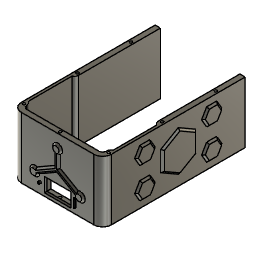
teslacoil assembly v1 (Autodesk Fusion 360 archive; units mm, degrees)
design "walls"
Autodesk Fusion 360 part; units mm, degrees
(part 1 of 3)
sketch "Sketch1" plane through (0, 0, 0) normal (0, 0, 1) x (1, 0, 0)
  line L0 (41.5, 125) -> (-41.5, 125)
  arc A0 (-41.5, 125) -> (-51.5, 115) centre (-41.5, 115) ccw
  line L1 (-51.5, 115) -> (-51.5, -130)
  arc A1 (51.5, 115) -> (41.5, 125) centre (41.5, 115) ccw
  line L2 (51.5, -130) -> (51.5, 115)
  line L3 (-41.5, -140) -> (41.5, -140)
  arc A2 (41.5, -140) -> (51.5, -130) centre (41.5, -130) ccw
  arc A3 (-51.5, -130) -> (-41.5, -140) centre (-41.5, -130) ccw
  line L4 (0, 125) -> (0, 122)
  line L5 (-51.5, 115) -> (-48.5, 115)
  circle A4 centre (-48.5, 115) radius 1.5
  circle A5 centre (0, 122) radius 1.5
  circle A6 centre (-48.5, -7.5) radius 1.5
  circle A7 centre (-48.5, 53.75) radius 1.5
  circle A8 centre (-48.5, -130) radius 1.5
  circle A9 centre (-48.5, -68.75) radius 1.5
  circle A10 centre (-48.5, -7.5) radius 1.5
  circle A11 centre (48.5, 115) radius 1.5
  circle A12 centre (48.5, 53.75) radius 1.5
  circle A13 centre (48.5, -7.5) radius 1.5
  circle A14 centre (48.5, -68.75) radius 1.5
  circle A15 centre (48.5, -130) radius 1.5
  line L6 (0, -140) -> (0, -137)
  circle A16 centre (0, -137) radius 1.5
  arc A17 (-45.5, -130) -> (-41.5, -134) centre (-41.5, -130) ccw
  line L7 (-41.5, -134) -> (41.5, -134)
  arc A18 (41.5, -134) -> (45.5, -130) centre (41.5, -130) ccw
  arc A19 (45.5, 115) -> (41.5, 119) centre (41.5, 115) ccw
  line L8 (41.5, 119) -> (-41.5, 119)
  line L9 (-48.5, -99.375) -> (-48.5, -75)
  line L10 (-48.5, -99.375) -> (-48.5, -125)
  line L11 (-45.5, 115) -> (-45.5, -75)
  line L12 (-45.5, -125) -> (-45.5, -130)
  line L13 (45.5, -130) -> (45.5, -125)
  line L14 (45.5, -75) -> (45.5, 115)
  line L15 (-48.5, -75) -> (-45.5, -75)
  line L16 (45.5, -75) -> (48.5, -75)
  line L17 (-48.5, -125) -> (-45.5, -125)
  line L18 (45.5, -125) -> (48.5, -125)
  line L19 (-48.5, -75) -> (-48.5, -125)
  line L20 (48.5, -75) -> (48.5, -125)
  arc A20 (-41.5, 119) -> (-45.5, 115) centre (-41.5, 115) ccw
  dimension "d1" = 3
  dimension "d3" = 3
  dimension "d4" = 3
  dimension "d5" = 3
  dimension "d7" = 3
  dimension "d8" = 3
  dimension "d9" = 3
  dimension "d10" = 3
  constraint midpoint L0 L4.start
  constraint perpendicular L0 L4
  constraint coincident L5.end A4.centre
  constraint coincident L4.end A5.centre
  constraint symmetric L4 A4 A11
  constraint symmetric L4 A7 A12
  constraint symmetric L4 A8 A15
  constraint symmetric L4 A9 A14
  constraint symmetric L4 A10 A13
  constraint midpoint L3 L6.start
  constraint perpendicular L3 L6
  constraint coincident L6.end A16.centre
  constraint perpendicular L10 L15
  constraint concentric A3 A17
  constraint concentric A2 A18
  constraint concentric A1 A19
  constraint tangent L7 A18
  constraint tangent A17 L7
  constraint tangent A17 L11
  constraint tangent A19 L13
  constraint tangent A18 L13
  constraint tangent A19 L8
  constraint collinear L11 L12
  constraint coincident L13.end L17
  constraint coincident L14.start L15
  constraint collinear L13 L14
  constraint collinear L15 L16
  constraint collinear L17 L18
  constraint symmetric L4 A19.start L11.start
  constraint symmetric L4 A19.end L8.end
  constraint symmetric L4 A19 A20
  measures "d1" distance of L4.start L4.end
  measures "d3" distance of A0.end L5.end
  measures "d4" diameter of A4
  measures "d5" diameter of A5
  measures "d7" diameter of A6
  measures "d8" diameter of A7
  measures "d9" distance of L6.start L6.end
  measures "d10" diameter of A16
extrude "Extrude1" add sketch "Sketch1" along normal blind 70
fillet "Fillet1" radius 5 4 edges at (45.5, -125, 35) (45.5, -75, 35) (-45.5, -75, 35) (-45.5, -125, 35)
sketch "Sketch2" plane through (0, 0, 70) normal (0, 0, 1) x (-1, 0, 0)
  arc A0 (45.5, 129.5826) -> (48.5, 125) centre (50.5, 129.5826) ccw
  line L0 (48.5, 125) -> (48.5, 75)
  arc A1 (48.5, 75) -> (45.5, 70.4174) centre (50.5, 70.4174) ccw
  line L1 (45.5, 70.4174) -> (45.5, -115)
  arc A2 (41.5, -119) -> (45.5, -115) centre (41.5, -115) ccw
  line L2 (41.5, -119) -> (-41.5, -119)
  arc A3 (-45.5, -115) -> (-41.5, -119) centre (-41.5, -115) ccw
  line L3 (-45.5, -115) -> (-45.5, 70.4174)
  arc A4 (-45.5, 70.4174) -> (-48.5, 75) centre (-50.5, 70.4174) ccw
  line L4 (-48.5, 75) -> (-48.5, 125)
  arc A5 (-48.5, 125) -> (-45.5, 129.5826) centre (-50.5, 129.5826) ccw
  line L5 (-45.5, 129.5826) -> (-45.5, 130)
  arc A6 (-41.5, 134) -> (-45.5, 130) centre (-41.5, 130) ccw
  line L6 (-41.5, 134) -> (41.5, 134)
  arc A7 (45.5, 130) -> (41.5, 134) centre (41.5, 130) ccw
  line L7 (45.5, 130) -> (45.5, 129.5826)
  circle A8 centre (48.5, -115) radius 1.5
  circle A9 centre (0, 137) radius 1.5
  circle A10 centre (0, -122) radius 1.5
  circle A11 centre (-48.5, 68.75) radius 1.5
  circle A12 centre (48.5, 130) radius 1.5
  circle A13 centre (-48.5, -115) radius 1.5
  circle A14 centre (-48.5, 130) radius 1.5
  circle A15 centre (48.5, 7.5) radius 1.5
  circle A16 centre (48.5, -53.75) radius 1.5
  circle A17 centre (-48.5, -53.75) radius 1.5
  circle A18 centre (-48.5, 7.5) radius 1.5
  circle A19 centre (48.5, 68.75) radius 1.5
  arc A20 (51.5, 130) -> (41.5, 140) centre (41.5, 130) ccw
  line L8 (41.5, 140) -> (-41.5, 140)
  arc A21 (-41.5, 140) -> (-51.5, 130) centre (-41.5, 130) ccw
  line L9 (-51.5, 130) -> (-51.5, -115)
  arc A22 (-51.5, -115) -> (-41.5, -125) centre (-41.5, -115) ccw
  line L10 (-41.5, -125) -> (41.5, -125)
  arc A23 (41.5, -125) -> (51.5, -115) centre (41.5, -115) ccw
  line L11 (51.5, -115) -> (51.5, 130)
  line L12 (48.5, -53.75) -> (48.5, 7.5)
  line L13 (-48.5, -53.75) -> (-48.5, 7.5)
  line L14 (48.5, -23.125) -> (-48.5, -23.125)
  line L15 (51.5, -23.125) -> (48.5, -23.125)
  line L16 (-48.5, -23.125) -> (-56, -23.125)
  constraint coincident A16.centre L12.start
  constraint coincident A15.centre L12.end
  constraint coincident A17.centre L13.start
  constraint coincident A18.centre L13.end
  constraint midpoint L12 L14.start
  constraint midpoint L13 L14.end
  constraint coincident L11 L15.start
  constraint perpendicular L12 L15
  constraint perpendicular L9 L16
extrude "Extrude2" cut sketch "Sketch2" against normal blind 80 contours L1 A2 L2 A3 L3 L9 A22 L10 A23 L11 L14 L15 L16
sketch "Sketch3" plane through (51.5, 0, 0) normal (1, 0, 0) x (0, 1, 0)
  line L0 (23.125, 0) -> (23.125, 70)
  line L1 (23.125, 70) -> (-130, 70)
  line L2 (-130, 70) -> (-130, 0)
  line L3 (-130, 0) -> (23.125, 0)
  line L4 (-53.4375, 70) -> (-53.4375, 0)
  line L5 (23.125, 35) -> (-130, 35)
  line L6 (-53.4375, 35) -> (-130, 70)
  line L7 (-53.4375, 35) -> (-130, 0)
  line L8 (-53.4375, 35) -> (23.125, 0)
  line L9 (-53.4375, 35) -> (23.125, 70)
  line L10 (-85.9452, 42.5) -> (-80.1717, 52.5)
  line L11 (-80.1717, 52.5) -> (-85.9452, 62.5)
  line L12 (-85.9452, 62.5) -> (-97.4923, 62.5)
  line L13 (-97.4923, 62.5) -> (-103.2658, 52.5)
  line L14 (-103.2658, 52.5) -> (-97.4923, 42.5)
  line L15 (-97.4923, 42.5) -> (-85.9452, 42.5)
  line L16 (-85.9452, 7.5) -> (-97.4923, 7.5)
  line L17 (-80.1717, 17.5) -> (-85.9452, 7.5)
  line L18 (-85.9452, 27.5) -> (-80.1717, 17.5)
  line L19 (-97.4923, 27.5) -> (-85.9452, 27.5)
  line L20 (-103.2658, 17.5) -> (-97.4923, 27.5)
  line L21 (-97.4923, 7.5) -> (-103.2658, 17.5)
  line L22 (-9.3827, 27.5) -> (-20.9298, 27.5)
  line L23 (-20.9298, 27.5) -> (-26.7033, 17.5)
  line L24 (-26.7033, 17.5) -> (-20.9298, 7.5)
  line L25 (-20.9298, 7.5) -> (-9.3827, 7.5)
  line L26 (-9.3827, 7.5) -> (-3.6092, 17.5)
  line L27 (-3.6092, 17.5) -> (-9.3827, 27.5)
  line L28 (-3.6092, 52.5) -> (-9.3827, 42.5)
  line L29 (-9.3827, 42.5) -> (-20.9298, 42.5)
  line L30 (-20.9298, 42.5) -> (-26.7033, 52.5)
  line L31 (-26.7033, 52.5) -> (-20.9298, 62.5)
  line L32 (-20.9298, 62.5) -> (-9.3827, 62.5)
  line L33 (-9.3827, 62.5) -> (-3.6092, 52.5)
  line L34 (-33.4375, 46.547) -> (-53.4375, 58.094)
  line L35 (-53.4375, 58.094) -> (-73.4375, 46.547)
  line L36 (-73.4375, 46.547) -> (-73.4375, 23.453)
  line L37 (-73.4375, 23.453) -> (-53.4375, 11.906)
  line L38 (-53.4375, 11.906) -> (-33.4375, 23.453)
  line L39 (-33.4375, 23.453) -> (-33.4375, 46.547)
  point P0 (-91.7188, 52.5)
  point P1 (-53.4375, 35)
  dimension "d18" = 10
  dimension "d19" = 20
  constraint midpoint L1 L4.start
  constraint midpoint L3 L4.end
  constraint midpoint L0 L5.start
  constraint midpoint L2 L5.end
  constraint midpoint L4 P1
  constraint coincident L1.end L2.start
  constraint coincident L2.end L3.start
  constraint coincident L0.start L3.end
  constraint coincident L0.end L1.start
  constraint midpoint L6 P0
  constraint symmetric L5 L10.start L18.start
  constraint symmetric L5 L10.end L17.start
  constraint symmetric L5 L11.end L16.start
  constraint symmetric L5 L12.end L16.end
  constraint symmetric L5 L13.end L20.start
  constraint symmetric L5 L14.end L19.start
  constraint symmetric L4 L10.start L29.end
  constraint symmetric L4 L10.end L30.end
  constraint symmetric L4 L11.end L31.end
  constraint symmetric L4 L12.end L32.end
  constraint symmetric L4 L13.end L28.start
  constraint symmetric L4 L14.end L28.end
  constraint symmetric L4 L16.start L24.end
  constraint symmetric L4 L16.end L25.end
  constraint symmetric L4 L17.start L23.end
  constraint symmetric L4 L18.start L22.end
  constraint symmetric L4 L19.start L22.start
  constraint symmetric L4 L20.start L26.end
  constraint coincident P1 L6.start
  measures "d18" distance of P0 L15
  measures "d19" distance of P1 L39
extrude "Extrude3" add sketch "Sketch3" along normal blind 2 contours L8 L23 L24 L25 L26 | L8 L22 L23 L26 L27 | L5 L8 L39 | L5 L9 L39 | L4 L7 L36 L37 | L4 L8 L38 L39 | L9 L28 L29 L30 L33 | L9 L30 L31 L32 L33 | L4 L6 L35 L36 | L5 L7 L36 | L5 L6 L36 | L4 L9 L34 L39 | L7 L18 L19 L20 L21 | L7 L16 L17 L18 L21 | L6 L10 L11 L12 L13 | L6 L10 L13 L14 L15
chamfer "Chamfer1" distance 2 angle 45 30 edges at (53.5, -63.4375, 52.3205) (53.5, -43.4375, 52.3205) (53.5, -33.4375, 35) (53.5, -43.4375, 17.6795) (53.5, -63.4375, 17.6795) (53.5, -73.4375, 35) (53.5, -91.7188, 42.5) (53.5, -83.0585, 57.5) (53.5, -100.379, 57.5) (53.5, -91.7188, 62.5) (53.5, -100.379, 47.5) (53.5, -100.379, 22.5) (53.5, -83.0585, 22.5) (53.5, -91.7188, 27.5) (53.5, -100.379, 12.5) (53.5, -91.7188, 7.5) (53.5, -83.0585, 12.5) (53.5, -83.0585, 47.5) (53.5, -15.1563, 62.5) (53.5, -6.496, 57.5) (53.5, -6.496, 47.5) (53.5, -15.1563, 42.5) (53.5, -23.8165, 47.5) (53.5, -23.8165, 57.5) (53.5, -23.8165, 22.5) (53.5, -23.8165, 12.5) (53.5, -15.1563, 7.5) (53.5, -6.496, 12.5) (53.5, -15.1563, 27.5) (53.5, -6.496, 22.5)
sketch "Sketch4" plane through (-51.5, 0, 0) normal (-1, 0, 0) x (0, -1, 0)
  line L0 (-23.125, 70) -> (-23.125, 0)
  line L1 (-23.125, 0) -> (130, 0)
  line L2 (130, 0) -> (130, 70)
  line L3 (130, 70) -> (-23.125, 70)
  line L4 (9.3827, 42.5) -> (20.9298, 42.5)
  line L5 (20.9298, 27.5) -> (26.7033, 17.5)
  line L6 (20.9298, 7.5) -> (9.3827, 7.5)
  line L7 (97.4923, 62.5) -> (103.2658, 52.5)
  line L8 (85.9452, 7.5) -> (97.4923, 7.5)
  line L9 (53.4375, 58.094) -> (33.4375, 46.547)
  line L10 (85.9452, 42.5) -> (80.1717, 52.5)
  line L11 (97.4923, 7.5) -> (103.2658, 17.5)
  line L12 (73.4375, 46.547) -> (53.4375, 58.094)
  line L13 (33.4375, 46.547) -> (33.4375, 23.453)
  line L14 (20.9298, 42.5) -> (26.7033, 52.5)
  line L15 (53.4375, 70) -> (53.4375, 0)
  line L16 (73.4375, 23.453) -> (73.4375, 46.547)
  line L17 (-23.125, 0) -> (130, 0)
  line L18 (53.4375, 35) -> (-23.125, 70)
  line L19 (53.4375, 11.906) -> (73.4375, 23.453)
  line L20 (9.3827, 7.5) -> (3.6092, 17.5)
  line L21 (103.2658, 17.5) -> (97.4923, 27.5)
  line L22 (85.9452, 62.5) -> (97.4923, 62.5)
  line L23 (85.9452, 27.5) -> (80.1717, 17.5)
  line L24 (-23.125, 70) -> (-23.125, 0)
  line L25 (103.2658, 52.5) -> (97.4923, 42.5)
  line L26 (9.3827, 27.5) -> (20.9298, 27.5)
  line L27 (3.6092, 52.5) -> (9.3827, 42.5)
  line L28 (80.1717, 52.5) -> (85.9452, 62.5)
  line L29 (53.4375, 35) -> (-23.125, 0)
  line L30 (97.4923, 27.5) -> (85.9452, 27.5)
  line L31 (80.1717, 17.5) -> (85.9452, 7.5)
  line L32 (53.4375, 35) -> (130, 70)
  line L33 (26.7033, 52.5) -> (20.9298, 62.5)
  line L34 (33.4375, 23.453) -> (53.4375, 11.906)
  line L35 (20.9298, 62.5) -> (9.3827, 62.5)
  line L36 (9.3827, 62.5) -> (3.6092, 52.5)
  line L37 (53.4375, 35) -> (130, 0)
  line L38 (130, 35) -> (-23.125, 35)
  line L39 (130, 0) -> (130, 70)
  line L40 (26.7033, 17.5) -> (20.9298, 7.5)
  line L41 (3.6092, 17.5) -> (9.3827, 27.5)
  line L42 (97.4923, 42.5) -> (85.9452, 42.5)
  line L43 (130, 70) -> (-23.125, 70)
  point P0 (15.1562, 52.5)
  point P1 (106.875, 0)
  point P2 (53.4375, 35)
  dimension "d23" = 10
  dimension "d24" = 20
  constraint midpoint L15.start L43
  constraint midpoint L15.end L17
  constraint midpoint L38.start L39
  constraint midpoint L38.end L24
  constraint midpoint P2 L15
  constraint coincident L0.start L3.end
  constraint coincident L0.end L1.start
  constraint coincident L1.end L2.start
  constraint coincident L2.end L3.start
  constraint midpoint P0 L18
  constraint symmetric L4.end L5.start L38
  constraint symmetric L14.end L5.end L38
  constraint symmetric L33.end L6.start L38
  constraint symmetric L35.end L6.end L38
  constraint symmetric L27.start L20.end L38
  constraint symmetric L4.start L26.start L38
  constraint symmetric L10.start L4.end L15
  constraint symmetric L10.end L14.end L15
  constraint symmetric L22.start L33.end L15
  constraint symmetric L7.start L35.end L15
  constraint symmetric L7.end L27.start L15
  constraint symmetric L25.end L4.start L15
  constraint symmetric L8.start L6.start L15
  constraint symmetric L8.end L6.end L15
  constraint symmetric L23.end L5.end L15
  constraint symmetric L23.start L5.start L15
  constraint symmetric L21.end L26.start L15
  constraint symmetric L11.end L20.end L15
  constraint coincident P2 L18.start
  measures "d23" distance of P0 L4
  measures "d24" distance of P2 L16
extrude "Extrude4" add sketch "Sketch4" along normal blind 2 contours L14 L18 L33 L35 L36 | L4 L14 L18 L27 L36 | L13 L29 L38 | L13 L18 L38 | L9 L13 L15 L18 | L12 L15 L16 L32 | L5 L6 L20 L29 L40 | L5 L20 L26 L29 L41 | L13 L15 L29 L34 | L15 L16 L19 L37 | L16 L37 L38 | L16 L32 L38 | L7 L10 L22 L28 L32 | L7 L10 L25 L32 L42 | L11 L21 L23 L30 L37 | L8 L11 L23 L31 L37
chamfer "Chamfer2" distance 2 angle 45 30 edges at (-53.5, -43.4375, 52.3205) (-53.5, -63.4375, 52.3205) (-53.5, -83.0585, 57.5) (-53.5, -91.7188, 62.5) (-53.5, -100.379, 57.5) (-53.5, -100.379, 47.5) (-53.5, -91.7188, 42.5) (-53.5, -83.0585, 47.5) (-53.5, -91.7188, 27.5) (-53.5, -83.0585, 22.5) (-53.5, -100.379, 22.5) (-53.5, -100.379, 12.5) (-53.5, -91.7188, 7.5) (-53.5, -83.0585, 12.5) (-53.5, -23.8165, 12.5) (-53.5, -15.1562, 7.5) (-53.5, -6.496, 12.5) (-53.5, -6.496, 22.5) (-53.5, -15.1562, 27.5) (-53.5, -23.8165, 22.5) (-53.5, -33.4375, 35) (-53.5, -43.4375, 17.6795) (-53.5, -73.4375, 35) (-53.5, -63.4375, 17.6795) (-53.5, -15.1562, 42.5) (-53.5, -23.8165, 47.5) (-53.5, -23.8165, 57.5) (-53.5, -15.1562, 62.5) (-53.5, -6.496, 57.5) (-53.5, -6.496, 47.5)
sketch "Sketch5" plane through (0, -140, 0) normal (0, -1, 0) x (1, 0, 0)
  line L0 (-41.5, 0) -> (41.5, 0)
  line L1 (41.5, 0) -> (41.5, 70)
  line L2 (41.5, 70) -> (-41.5, 70)
  line L3 (-41.5, 70) -> (-41.5, 0)
  line L4 (0, 70) -> (0, 0)
  line L5 (0, 35) -> (-25.9808, 20)
  circle A0 centre (-25.9808, 20) radius 5.5
  line L6 (-1.5, 37.5981) -> (-27.4808, 22.5981)
  circle A1 centre (0, 55) radius 5.5
  line L7 (-3, 70) -> (-3, 0)
  line L8 (1.5, 32.4019) -> (-24.4808, 17.4019)
  line L9 (3, 70) -> (3, 0)
  line L10 (1.5, 37.5981) -> (27.4808, 22.5981)
  line L11 (0, 35) -> (25.9808, 20)
  circle A2 centre (25.9808, 20) radius 5.5
  line L12 (-1.5, 32.4019) -> (24.4808, 17.4019)
  dimension "d28" = 120
  dimension "d29" = 30
  dimension "d30" = 11
  dimension "d31" = 3
  dimension "d32" = 11
  dimension "d33" = 3
  dimension "d34" = -3
  dimension "d35" = -3
  constraint midpoint L2 L4.start
  constraint coincident L4.end origin
  constraint midpoint L4 L5.start
  constraint coincident L5.end A0.centre
  constraint coincident L4 A1.centre
  constraint symmetric L4 L5.start L11.start
  constraint symmetric L4 L5.end L11.end
  constraint symmetric L4 A0 A2
  constraint symmetric L4 L6.start L10.start
  constraint symmetric L4 L6.end L10.end
  constraint symmetric L4 L8.start L12.start
  constraint symmetric L4 L8.end L12.end
  measures "d28" angle of L4 L5
  measures "d29" distance of L5.start L5.end
  measures "d30" diameter of A0
  measures "d32" diameter of A1
extrude "Extrude5" add sketch "Sketch5" along normal blind 2 contours L5 A0 L7 L8 | L4 L5 L7 L8 | L4 L9 L11 L12 | L4 L5 A1 L7 | L5 A0 L6 L7 | A0 | A1 L7 | L4 A1 L7 | L9 L11 A2 L12 | L4 A1 L9 L11 | L4 A1 L9 | L9 L10 L11 A2 | A2 | A1 L9
chamfer "Chamfer3" distance 2 angle 45 9 edges at (-13.2443, -142, 30.8175) (-10.2443, -142, 25.6214) (-30.7439, -142, 17.25) (30.7439, -142, 17.25) (10.2443, -142, 25.6214) (13.2443, -142, 30.8175) (3, -142, 43.5611) (-3, -142, 43.5611) (0, -142, 60.5)
sketch "Sketch6" plane through (0, -140, 0) normal (0, -1, 0) x (1, 0, 0)
  line L0 (0, 31.5359) -> (-20.4886, 19.7068)
  arc A0 (-23.4886, 24.903) -> (-20.4886, 19.7068) centre (-25.9808, 20) ccw
  line L1 (-23.4886, 24.903) -> (-3, 36.7321)
  line L2 (-3, 36.7321) -> (-3, 50.3902)
  arc A1 (3, 50.3902) -> (-3, 50.3902) centre (0, 55) ccw
  line L3 (3, 50.3902) -> (3, 36.7321)
  line L4 (3, 36.7321) -> (23.4886, 24.903)
  arc A2 (20.4886, 19.7068) -> (23.4886, 24.903) centre (25.9808, 20) ccw
  line L5 (20.4886, 19.7068) -> (0, 31.5359)
  line L6 (-41.5, 0) -> (41.5, 0)
  line L7 (41.5, 0) -> (41.5, 70)
  line L8 (41.5, 70) -> (-41.5, 70)
  line L9 (-41.5, 70) -> (-41.5, 0)
  line L10 (0, 0) -> (0, 5)
  line L11 (0, 5) -> (13.7, 5)
  line L12 (0, 5) -> (-13.7, 5)
  line L13 (13.7, 5) -> (13.7, 18.2)
  line L14 (-13.7, 5) -> (-13.7, 18.2)
  line L15 (13.7, 18.2) -> (-13.7, 18.2)
  dimension "d39" = 5
  dimension "d40" = 13.7
  dimension "d41" = 13.7
  dimension "d42" = 13.2
  dimension "d43" = 13.2
  constraint coincident L10.start origin
  constraint perpendicular L6 L10
  constraint perpendicular L10 L11
  constraint perpendicular L10 L12
  constraint perpendicular L11 L13
  constraint perpendicular L12 L14
  measures "d39" distance of L10.start L10.end
  measures "d40" distance of L10.end L11.end
  measures "d41" distance of L10.end L12.end
  measures "d42" distance of L11.end L13.end
  measures "d43" distance of L12.end L14.end
extrude "Extrude6" cut sketch "Sketch6" against normal blind 50 contours L11 L12 L13 L14 L15
chamfer "Chamfer4" distance 1.5 angle 45 4 edges at (0, -140, 5) (13.7, -140, 11.6) (0, -140, 18.2) (-13.7, -140, 11.6)
sketch "Sketch7" plane through (0, -140, 0) normal (0, -1, 0) x (1, 0, 0)
  line L0 (-41.5, 0) -> (41.5, 0)
  line L1 (41.5, 0) -> (41.5, 70)
  line L2 (41.5, 70) -> (-41.5, 70)
  line L3 (-41.5, 70) -> (-41.5, 0)
  line L4 (0, 31.5359) -> (-20.4886, 19.7068)
  arc A0 (-23.4886, 24.903) -> (-20.4886, 19.7068) centre (-25.9808, 20) ccw
  line L5 (-23.4886, 24.903) -> (-3, 36.7321)
  line L6 (-3, 36.7321) -> (-3, 50.3902)
  arc A1 (3, 50.3902) -> (-3, 50.3902) centre (0, 55) ccw
  line L7 (3, 50.3902) -> (3, 36.7321)
  line L8 (3, 36.7321) -> (23.4886, 24.903)
  arc A2 (20.4886, 19.7068) -> (23.4886, 24.903) centre (25.9808, 20) ccw
  line L9 (20.4886, 19.7068) -> (0, 31.5359)
  line L10 (-15.2, 19.7) -> (15.2, 19.7)
  line L11 (15.2, 19.7) -> (15.2, 3.5)
  line L12 (15.2, 3.5) -> (-15.2, 3.5)
  line L13 (-15.2, 3.5) -> (-15.2, 19.7)
  line L14 (15.2, 3.5) -> (15.2, 19.7)
  line L15 (15.2, 11.6) -> (20.2, 11.6)
  line L16 (-15.2, 11.6) -> (-20.2, 11.6)
  line L17 (20.2, 11.6) -> (20.2, 7)
  line L18 (21, 7) -> (21, 16.2)
  arc A3 (21, 16.2) -> (19.4, 16.2) centre (20.2, 16.2) ccw
  line L19 (19.4, 16.2) -> (19.4, 7)
  arc A4 (19.4, 7) -> (21, 7) centre (20.2, 7) ccw
  line L20 (20.2, 7) -> (20.2, 16.2) construction
  circle A5 centre (-20.2, 11.6) radius 1.5
  dimension "d47" = 5
  dimension "d48" = 5
  dimension "d49" = 3
  constraint coincident L11.end L12.start
  constraint coincident L10.end L11.start
  constraint midpoint L11 L15.start
  constraint perpendicular L11 L15
  constraint midpoint L13 L16.start
  constraint perpendicular L13 L16
  constraint perpendicular L15 L17
  constraint tangent L18 A3
  constraint tangent A3 L19
  constraint parallel L18 L19
  constraint tangent L19 A4
  constraint tangent L18 A4
  constraint perpendicular L15 L20
  constraint coincident L17.end A4.centre
  constraint coincident L16.end A5.centre
  measures "d47" distance of L15.start L15.end
  measures "d48" distance of L16.start L16.end
  measures "d49" diameter of A5
extrude "Extrude7" add sketch "Sketch7" along normal blind 2 contours L18 A3 L19 A4 | A5
chamfer "Chamfer5" distance 0.75 angle 45 5 edges at (21, -142, 11.6) (20.2, -142, 17) (19.4, -142, 11.6) (20.2, -142, 6.2) (-21.5985, -142, 11.0576)

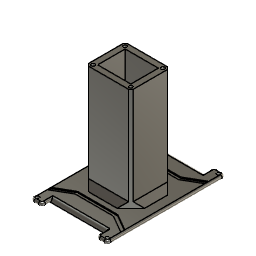
design "handle2"
Autodesk Fusion 360 part; units mm, degrees
sketch "Sketch1" plane through (0, 0, 0) normal (0, 0, 1) x (1, 0, 0)
  line L0 (0, 0) -> (-30.625, 0)
  line L1 (0, 0) -> (30.625, 0)
  line L2 (-30.625, 0) -> (-30.625, 97)
  line L3 (-30.625, 97) -> (30.625, 97)
  line L4 (30.625, 97) -> (30.625, 0)
  circle A0 centre (-30.625, 97) radius 1.5
  circle A1 centre (30.625, 97) radius 1.5
  circle A2 centre (-30.625, 0) radius 1.5
  circle A3 centre (30.625, 0) radius 1.5
  line L5 (0, -3) -> (33.625, -3)
  line L6 (33.625, 100) -> (33.625, -3)
  line L7 (-33.625, 100) -> (33.625, 100)
  line L8 (-33.625, -3) -> (-33.625, 100)
  line L9 (0, -3) -> (-33.625, -3)
  dimension "d1" = 30.625
  dimension "d2" = 30.625
  dimension "d3" = 97
  dimension "d4" = 61.25
  dimension "d5" = 3
  dimension "d6" = 3
  dimension "d7" = 3
  dimension "d8" = 3
  dimension "d9" = -3
  constraint coincident L0.start L1.start
  constraint horizontal L0
  constraint parallel L0 L1
  constraint perpendicular L0 L2
  constraint perpendicular L2 L3
  constraint coincident L2.end L3.start
  constraint coincident L3.end L4.start
  constraint coincident L0.end L2.start
  constraint coincident L1.end L4.end
  measures "d1" distance of L0.start L0.end
  measures "d2" distance of L0.start L1.end
  measures "d3" distance of L0.end L2.end
  measures "d4" distance of L2.end L3.end
  measures "d5" diameter of A0
  measures "d6" diameter of A1
  measures "d7" diameter of A2
  measures "d8" diameter of A3
extrude "Extrude1" add sketch "Sketch1" along normal blind 3 contours L0 L1 L2 L3 L4 A0 A1 A2 A3 | L5 L6 L7 L8 L9
sketch "Sketch2" plane through (0, 0, 3) normal (0, 0, 1) x (-1, 0, 0)
  circle A0 centre (30.625, 0) radius 1.5
  circle A1 centre (30.625, -97) radius 1.5
  circle A2 centre (-30.625, 0) radius 1.5
  circle A3 centre (-30.625, -97) radius 1.5
  line L0 (33.625, 3) -> (-33.625, 3)
  line L1 (-33.625, 3) -> (-33.625, -100)
  line L2 (-33.625, -100) -> (33.625, -100)
  line L3 (33.625, -100) -> (33.625, 3)
  line L4 (14.5, -60.5) -> (-14.5, -60.5)
  circle A4 centre (-16.5, -34.5) radius 1.5
  line L5 (14.5, -36.5) -> (14.5, -60.5)
  circle A5 centre (16.5, -62.5) radius 1.5
  line L6 (-17.5, -65.5) -> (17.5, -65.5)
  line L7 (-19.5, -33.5) -> (-19.5, -63.5)
  line L8 (17.5, -65.5) -> (19.5, -63.5)
  line L9 (19.5, -63.5) -> (19.5, -33.5)
  line L10 (17.5, -31.5) -> (-17.5, -31.5)
  circle A6 centre (-16.5, -62.5) radius 1.5
  line L11 (19.5, -33.5) -> (17.5, -31.5)
  line L12 (-17.5, -31.5) -> (-19.5, -33.5)
  line L13 (-14.5, -60.5) -> (-14.5, -36.5)
  circle A7 centre (16.5, -34.5) radius 1.5
  line L14 (-19.5, -63.5) -> (-17.5, -65.5)
  line L15 (-14.5, -36.5) -> (14.5, -36.5)
  line L16 (33.625, -48.5) -> (-33.625, -48.5)
  line L17 (0, -48.5) -> (0, -70)
  point P0 (0, -48.5)
  constraint midpoint L3 L16.start
  constraint midpoint L1 L16.end
  constraint midpoint L16 P0
  constraint perpendicular L16 L17
  measures "d28" angle of L0.end
extrude "Extrude2" add sketch "Sketch2" along normal blind 90 contours L5 L7 L9 L10 L11 L12 L13 L15 L16 | L4 L5 L6 L8 L9 L16 L17 | L4 L6 L7 L13 L14 L16 L17
sketch "Sketch3" plane through (0, 0, 3) normal (0, 0, 1) x (-1, 0, 0)
  line L0 (-14.5, -60.5) -> (14.5, -60.5)
  line L1 (14.5, -60.5) -> (14.5, -36.5)
  line L2 (14.5, -36.5) -> (-14.5, -36.5)
  line L3 (-14.5, -36.5) -> (-14.5, -60.5)
  line L4 (33.625, 3) -> (-33.625, 3)
  line L5 (-33.625, 3) -> (-33.625, -100)
  line L6 (-33.625, -100) -> (33.625, -100)
  line L7 (33.625, -100) -> (33.625, 3)
  circle A0 centre (-30.625, -97) radius 1.5
  circle A1 centre (-30.625, 0) radius 1.5
  circle A2 centre (30.625, -97) radius 1.5
  circle A3 centre (30.625, 0) radius 1.5
  line L8 (-19.5, -63.5) -> (-19.5, -33.5)
  line L9 (-19.5, -33.5) -> (-17.5, -31.5)
  line L10 (-17.5, -31.5) -> (17.5, -31.5)
  line L11 (17.5, -31.5) -> (19.5, -33.5)
  line L12 (19.5, -33.5) -> (19.5, -63.5)
  line L13 (19.5, -63.5) -> (17.5, -65.5)
  line L14 (17.5, -65.5) -> (-17.5, -65.5)
  line L15 (-17.5, -65.5) -> (-19.5, -63.5)
  line L16 (30.625, 0) -> (23.625, 0)
  line L17 (23.625, 3) -> (23.625, -5)
  line L18 (-30.625, 0) -> (-23.625, 0)
  line L19 (-23.625, 3) -> (-23.625, -5)
  line L20 (23.625, -5) -> (-23.625, -5)
  line L21 (33.625, -48.5) -> (56.2227, -48.5)
  line L22 (23.625, -92) -> (-23.625, -92)
  line L23 (33.625, -100) -> (-33.625, -100)
  line L24 (23.625, -100) -> (23.625, -92)
  line L25 (-23.625, -100) -> (-23.625, -92)
  line L26 (-30.625, -97) -> (-23.625, -97)
  line L27 (30.625, -97) -> (23.625, -97)
  point P0 (0, -97)
  dimension "d14" = 7
  dimension "d15" = 8
  dimension "d16" = 7
  dimension "d17" = 8
  constraint coincident A3.centre L16.start
  constraint parallel L4 L16
  constraint coincident L4 L17.start
  constraint perpendicular L16 L17
  constraint coincident A1.centre L18.start
  constraint perpendicular L5 L18
  constraint coincident L4 L19.start
  constraint perpendicular L18 L19
  constraint midpoint L7 L21.start
  constraint perpendicular L7 L21
  constraint symmetric origin L21 P0
  constraint symmetric L4.start L21 L6.end
  constraint symmetric L4.end L21 L5.end
  constraint symmetric A3.centre L21 A2.centre
  constraint symmetric L16.end L21 L27.end
  constraint symmetric L17.start L21 L24.start
  constraint symmetric L17.end L21 L22.start
  constraint symmetric A1.centre L21 A0.centre
  constraint symmetric L18.end L21 L26.end
  constraint symmetric L19.start L21 L25.start
  constraint symmetric L19.end L21 L22.end
  measures "d14" distance of A3.centre L16.end
  measures "d15" distance of L17.start L17.end
  measures "d16" distance of A1.centre L18.end
  measures "d17" distance of L19.start L19.end
extrude "Extrude3" cut sketch "Sketch3" against normal blind 5 contours L0 L1 L2 L3 | L4 L17 L19 L20 | L6 L22 L23 L24 L25
fillet "Fillet1" radius 3 2 edges at (0, 92, 3) (0, 5, 3)
fillet "Fillet2" radius 3 8 edges at (-23.625, -3, 1.5) (-33.625, -3, 1.5) (33.625, -3, 1.5) (23.625, -3, 1.5) (-33.625, 100, 1.5) (-23.625, 100, 1.5) (23.625, 100, 1.5) (33.625, 100, 1.5)
fillet "Fillet3" radius 1.5 36 edges at (23.625, 4, 3) (24.5037, -2.1213, 3) (28.625, -3, 3) (32.7463, -2.1213, 3) (33.625, 48.5, 3) (32.7463, 99.1213, 3) (28.625, 100, 3) (24.5037, 99.1213, 3) (23.625, 93, 3) (-23.625, 93, 3) (-24.5037, 99.1213, 3) (-28.625, 100, 3) (-32.7463, 99.1213, 3) (-33.625, 48.5, 3) (-32.7463, -2.1213, 3) (-28.625, -3, 3) (-24.5037, -2.1213, 3) (-23.625, 4, 3) (23.625, 94.5, 0) (24.5037, 99.1213, 0) (28.625, 100, 0) (32.7463, 99.1213, 0) (33.625, 48.5, 0) (32.7463, -2.1213, 0) (28.625, -3, 0) (24.5037, -2.1213, 0) (23.625, 2.5, 0) (-23.625, 2.5, 0) (-24.5037, -2.1213, 0) (-28.625, -3, 0) (-32.7463, -2.1213, 0) (-33.625, 48.5, 0) (-32.7463, 99.1213, 0) (-28.625, 100, 0) (-24.5037, 99.1213, 0) (-23.625, 94.5, 0)
sketch "Sketch4" plane through (0, 0, 3) normal (0, 0, 1) x (-1, 0, 0)
  line L0 (25.125, -8) -> (-25.125, -8)
  line L1 (-25.125, -8) -> (-25.125, 0)
  arc A0 (-25.125, 0) -> (-26.625, 1.5) centre (-26.625, 0) ccw
  line L2 (-26.625, 1.5) -> (-30.625, 1.5)
  arc A1 (-32.125, 0) -> (-30.625, 1.5) centre (-30.625, 0) ccw
  line L3 (-32.125, 0) -> (-32.125, -97)
  arc A2 (-30.625, -98.5) -> (-32.125, -97) centre (-30.625, -97) ccw
  line L4 (-30.625, -98.5) -> (-26.625, -98.5)
  arc A3 (-26.625, -98.5) -> (-25.125, -97) centre (-26.625, -97) ccw
  line L5 (-25.125, -97) -> (-25.125, -89)
  line L6 (-25.125, -89) -> (25.125, -89)
  line L7 (25.125, -89) -> (25.125, -97)
  arc A4 (25.125, -97) -> (26.625, -98.5) centre (26.625, -97) ccw
  line L8 (26.625, -98.5) -> (30.625, -98.5)
  arc A5 (32.125, -97) -> (30.625, -98.5) centre (30.625, -97) ccw
  line L9 (32.125, -97) -> (32.125, 0)
  arc A6 (30.625, 1.5) -> (32.125, 0) centre (30.625, 0) ccw
  line L10 (30.625, 1.5) -> (26.625, 1.5)
  arc A7 (26.625, 1.5) -> (25.125, 0) centre (26.625, 0) ccw
  line L11 (25.125, 0) -> (25.125, -8)
  line L12 (-19.5, -63.5) -> (-19.5, -33.5)
  line L13 (-19.5, -33.5) -> (-17.5, -31.5)
  line L14 (-17.5, -31.5) -> (17.5, -31.5)
  line L15 (17.5, -31.5) -> (19.5, -33.5)
  line L16 (19.5, -33.5) -> (19.5, -63.5)
  line L17 (19.5, -63.5) -> (17.5, -65.5)
  line L18 (17.5, -65.5) -> (-17.5, -65.5)
  line L19 (-17.5, -65.5) -> (-19.5, -63.5)
  line L20 (0, -75) -> (17.5, -75)
  line L21 (17.5, -75) -> (43.5708, -90.052)
  line L22 (17.5, -75) -> (47.604, -75) construction
  line L23 (32.125, -48.5) -> (46.4762, -48.5)
  line L24 (-17.5, -75) -> (-43.5708, -90.052)
  line L25 (0, -75) -> (-17.5, -75)
  line L26 (16.6962, -78) -> (42.0708, -92.6501)
  line L27 (0, -78) -> (16.6962, -78)
  line L28 (0, -78) -> (-16.6962, -78)
  line L29 (-16.6962, -78) -> (-42.0708, -92.6501)
  line L30 (16.6962, -19) -> (42.0708, -4.3499)
  line L31 (17.5, -22) -> (43.5708, -6.948)
  line L32 (0, -22) -> (17.5, -22)
  line L33 (0, -19) -> (16.6962, -19)
  line L34 (-16.6962, -19) -> (-42.0708, -4.3499)
  line L35 (-17.5, -22) -> (-43.5708, -6.948)
  line L36 (0, -22) -> (-17.5, -22)
  line L37 (0, -19) -> (-16.6962, -19)
  line L38 (33.625, 0) -> (32.125, 0)
  line L39 (32.125, 0) -> (32.125, -97)
  line L40 (32.125, -97) -> (33.625, -97)
  line L41 (32.125, -97) -> (32.125, 0)
  line L42 (32.125, -97) -> (33.625, -97)
  arc A8 (30.625, -98.5) -> (32.125, -97) centre (30.625, -97) ccw
  line L43 (30.625, -100) -> (30.625, -98.5)
  arc A9 (30.625, -98.5) -> (32.125, -97) centre (30.625, -97) ccw
  line L44 (30.625, -100) -> (30.625, -98.5)
  line L45 (30.625, -98.5) -> (26.625, -98.5)
  line L46 (26.625, -98.5) -> (26.625, -100)
  line L47 (26.625, -98.5) -> (30.625, -98.5)
  line L48 (26.625, -98.5) -> (26.625, -100)
  arc A10 (25.125, -97) -> (26.625, -98.5) centre (26.625, -97) ccw
  line L49 (23.625, -97) -> (25.125, -97)
  arc A11 (25.125, -97) -> (26.625, -98.5) centre (26.625, -97) ccw
  line L50 (23.625, -97) -> (25.125, -97)
  line L51 (25.125, -97) -> (25.125, -89)
  spline S0 degree 3 poles (23.625, -91.5981) (23.625, -91.4847) (23.6653, -91.3409) (23.8021, -91.0199) (23.898, -90.8428) (24.1441, -90.426) (24.329, -90.1444) (24.7236, -89.5673) (24.9329, -89.2716) (25.125, -89) knots 0.801784 0.801784 0.801784 0.801784 0.869795 0.869795 0.937806 0.937806 1.037599 1.037599 1.137392 1.137392 1.137392 1.137392
  spline S1 degree 3 poles (25.125, -92) (24.9363, -92) (24.7352, -92.0007) (24.3655, -91.9949) (24.197, -91.9873) (23.9239, -91.9469) (23.8064, -91.9096) (23.6572, -91.7856) (23.625, -91.6979) (23.625, -91.5981) knots 0.568638 0.568638 0.568638 0.568638 0.625237 0.625237 0.681836 0.681836 0.741752 0.741752 0.801668 0.801668 0.801668 0.801668
  line L52 (25.125, -92) -> (25.125, -97)
  line L53 (-25.125, -92) -> (25.125, -92)
  spline S2 degree 3 poles (25.125, -92) (24.9363, -92) (24.7352, -92.0007) (24.3655, -91.9949) (24.197, -91.9873) (23.9239, -91.9469) (23.8064, -91.9096) (23.6572, -91.7856) (23.625, -91.6979) (23.625, -91.5981) knots 0.568638 0.568638 0.568638 0.568638 0.625237 0.625237 0.681836 0.681836 0.741752 0.741752 0.801668 0.801668 0.801668 0.801668
  spline S3 degree 3 poles (23.625, -91.5981) (23.625, -91.4847) (23.6653, -91.3409) (23.8021, -91.0199) (23.898, -90.8428) (24.1441, -90.426) (24.329, -90.1444) (24.7236, -89.5673) (24.9329, -89.2716) (25.125, -89) knots 0.801784 0.801784 0.801784 0.801784 0.869795 0.869795 0.937806 0.937806 1.037599 1.037599 1.137392 1.137392 1.137392 1.137392
  line L54 (25.125, -89) -> (-25.125, -89)
  spline S4 degree 3 poles (-25.125, -89) (-24.9329, -89.2716) (-24.7236, -89.5673) (-24.329, -90.1444) (-24.1441, -90.426) (-23.898, -90.8428) (-23.8021, -91.0199) (-23.6653, -91.3409) (-23.625, -91.4847) (-23.625, -91.5981) knots 0 0 0 0 0.099793 0.099793 0.199586 0.199586 0.267597 0.267597 0.335608 0.335608 0.335608 0.335608
  spline S5 degree 3 poles (-23.625, -91.5981) (-23.625, -91.6979) (-23.6572, -91.7856) (-23.8064, -91.9096) (-23.9239, -91.9469) (-24.197, -91.9873) (-24.3655, -91.9949) (-24.7352, -92.0007) (-24.9363, -92) (-25.125, -92) knots 0.335608 0.335608 0.335608 0.335608 0.395524 0.395524 0.455441 0.455441 0.512039 0.512039 0.568638 0.568638 0.568638 0.568638
  line L55 (30.625, 1.5) -> (30.625, 3)
  arc A12 (32.125, 0) -> (30.625, 1.5) centre (30.625, 0) ccw
  line L56 (33.625, 0) -> (32.125, 0)
  arc A13 (32.125, 0) -> (30.625, 1.5) centre (30.625, 0) ccw
  line L57 (26.625, 3) -> (26.625, 1.5)
  line L58 (26.625, 1.5) -> (30.625, 1.5)
  line L59 (30.625, 1.5) -> (30.625, 3)
  line L60 (30.625, 1.5) -> (26.625, 1.5)
  line L61 (25.125, 0) -> (23.625, 0)
  arc A14 (26.625, 1.5) -> (25.125, 0) centre (26.625, 0) ccw
  line L62 (26.625, 3) -> (26.625, 1.5)
  arc A15 (26.625, 1.5) -> (25.125, 0) centre (26.625, 0) ccw
  spline S6 degree 3 poles (25.125, -8) (24.9329, -7.7284) (24.7236, -7.4327) (24.329, -6.8556) (24.1441, -6.574) (23.898, -6.1572) (23.8021, -5.9801) (23.6653, -5.6591) (23.625, -5.5153) (23.625, -5.4019) knots 0 0 0 0 0.099793 0.099793 0.199586 0.199586 0.267597 0.267597 0.335608 0.335608 0.335608 0.335608
  line L63 (25.125, -8) -> (25.125, 0)
  line L64 (25.125, 0) -> (23.625, 0)
  line L65 (25.125, 0) -> (25.125, -5)
  spline S7 degree 3 poles (23.625, -5.4019) (23.625, -5.3021) (23.6572, -5.2144) (23.8064, -5.0904) (23.9239, -5.0531) (24.197, -5.0127) (24.3655, -5.0051) (24.7352, -4.9993) (24.9363, -5) (25.125, -5) knots 0.335608 0.335608 0.335608 0.335608 0.395524 0.395524 0.455441 0.455441 0.512039 0.512039 0.568638 0.568638 0.568638 0.568638
  line L66 (25.125, -5) -> (-25.125, -5)
  spline S8 degree 3 poles (-25.125, -5) (-24.9363, -5) (-24.7352, -4.9993) (-24.3655, -5.0051) (-24.197, -5.0127) (-23.9239, -5.0531) (-23.8064, -5.0904) (-23.6572, -5.2144) (-23.625, -5.3021) (-23.625, -5.4019) knots 0.568638 0.568638 0.568638 0.568638 0.625237 0.625237 0.681836 0.681836 0.741752 0.741752 0.801668 0.801668 0.801668 0.801668
  spline S9 degree 3 poles (-23.625, -5.4019) (-23.625, -5.5153) (-23.6653, -5.6591) (-23.8021, -5.9801) (-23.898, -6.1572) (-24.1441, -6.574) (-24.329, -6.8556) (-24.7236, -7.4327) (-24.9329, -7.7284) (-25.125, -8) knots 0.801668 0.801668 0.801668 0.801668 0.869679 0.869679 0.93769 0.93769 1.037483 1.037483 1.137277 1.137277 1.137277 1.137277
  line L67 (-25.125, -8) -> (25.125, -8)
  spline S10 degree 3 poles (25.125, -8) (24.9329, -7.7284) (24.7236, -7.4327) (24.329, -6.8556) (24.1441, -6.574) (23.898, -6.1572) (23.8021, -5.9801) (23.6653, -5.6591) (23.625, -5.5153) (23.625, -5.4019) knots 0 0 0 0 0.099793 0.099793 0.199586 0.199586 0.267597 0.267597 0.335608 0.335608 0.335608 0.335608
  spline S11 degree 3 poles (23.625, -5.4019) (23.625, -5.3021) (23.6572, -5.2144) (23.8064, -5.0904) (23.9239, -5.0531) (24.197, -5.0127) (24.3655, -5.0051) (24.7352, -4.9993) (24.9363, -5) (25.125, -5) knots 0.335608 0.335608 0.335608 0.335608 0.395524 0.395524 0.455441 0.455441 0.512039 0.512039 0.568638 0.568638 0.568638 0.568638
  line L68 (-33.625, -97) -> (-32.125, -97)
  line L69 (-32.125, -97) -> (-32.125, 0)
  line L70 (-32.125, 0) -> (-33.625, 0)
  line L71 (-32.125, 0) -> (-32.125, -97)
  dimension "d27" = 17.5
  dimension "d28" = 30
  dimension "d29" = -3
  constraint horizontal L22
  constraint midpoint L9 L23.start
  constraint perpendicular L9 L23
  constraint symmetric L20.start L23 L32.start
  constraint symmetric L20.end L23 L31.start
  constraint symmetric L21.end L23 L31.end
  constraint symmetric L23 L24.start L35.start
  constraint symmetric L23 L24.end L35.end
  constraint symmetric L23 L20.start L32.start
  constraint symmetric L23 L26.start L30.start
  constraint symmetric L23 L26.end L30.end
  constraint symmetric L23 L27.start L33.start
  constraint symmetric L23 L28.end L34.start
  constraint symmetric L23 L29.end L34.end
  measures "d27" distance of L20.start L20.end
  measures "d28" angle of L21 L22
extrude "Extrude4" cut sketch "Sketch4" against normal blind 1 contours L3 L9 L30 L31 L32 L33 L34 L35 L36 L37 L39 L41 L69 L71 | L3 L9 L20 L21 L24 L25 L26 L27 L28 L29 L39 L41 L69 L71
chamfer "Chamfer1" distance 5 angle 45 4 edges at (0, 31.5, 3) (0, 65.5, 3) (19.5, 48.5, 3) (-19.5, 48.5, 3)

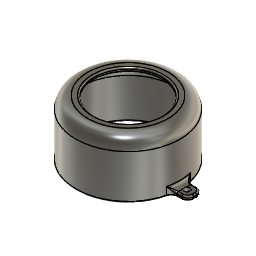
design "sheath"
Autodesk Fusion 360 part; units mm, degrees
sketch "Sketch1" plane through (0, 0, 0) normal (0, 0, 1) x (1, 0, 0)
  circle A0 centre (0, 0) radius 35
  circle A1 centre (0, 0) radius 32
  dimension "d1" = 70
  dimension "d2" = -3
  constraint coincident A0.centre A1.centre
  measures "d1" diameter of A0
extrude "Extrude1" add sketch "Sketch1" along normal blind 38
sketch "Sketch2" plane through (0, 0, 38) normal (0, 0, 1) x (-1, 0, 0)
  circle A0 centre (0, 0) radius 32
  circle A1 centre (0, 0) radius 35
  circle A2 centre (0, 0) radius 35
  circle A3 centre (0, 0) radius 23
  circle A4 centre (0, 0) radius 32
  dimension "d5" = 46
  constraint coincident A0.centre A1.centre
  constraint concentric A2 A4
  measures "d5" diameter of A3
extrude "Extrude2" add sketch "Sketch2" against normal blind 3 contours A0 A4
fillet "Fillet1" radius 8 1 edges at (-29.8345, -11.5717, 35)
fillet "Fillet2" radius 8 1 edges at (-32.6315, -12.6565, 38)
sketch "Sketch3" plane through (0, 0, 0) normal (0, 0, -1) x (1, 0, 0)
  circle A0 centre (0, 0) radius 32
  circle A1 centre (0, 0) radius 35
  line L0 (0, 0) -> (39.625, 0)
  circle A2 centre (39.625, 0) radius 2
  line L1 (35, 0) -> (45, 0)
  line L2 (45, 0) -> (45, -5)
  line L3 (45, -5) -> (34.641, -5)
  line L4 (45, 0) -> (45, 5)
  line L5 (45, 5) -> (34.641, 5)
  line L6 (0, 0) -> (0, -10)
  circle A3 centre (-39.625, 0) radius 2
  line L7 (-45, -5) -> (-34.641, -5)
  line L8 (-45, 0) -> (-45, -5)
  line L9 (-45, 0) -> (-45, 5)
  line L10 (-45, 5) -> (-34.641, 5)
  dimension "d12" = 39.625
  dimension "d13" = 4
  dimension "d14" = 10
  dimension "d15" = 5
  dimension "d16" = 5
  constraint coincident A0.centre A1.centre
  constraint horizontal L0
  constraint coincident L0.end A2.centre
  constraint coincident L0 L1.start
  constraint coincident A1 L1.start
  constraint parallel L0 L1
  constraint perpendicular L1 L2
  constraint coincident A1 L3.end
  constraint perpendicular L2 L3
  constraint perpendicular L1 L4
  constraint coincident A1 L5.end
  constraint perpendicular L4 L5
  constraint perpendicular L0 L6
  constraint symmetric A2 L6 A3
  constraint symmetric L1.end L6 L8.start
  constraint symmetric L2.end L6 L7.start
  constraint symmetric L3.end L6 L7.end
  constraint symmetric L4.end L6 L9.end
  constraint symmetric L5.end L6 L10.end
  measures "d12" distance of A0.centre L0.end
  measures "d13" diameter of A2
  measures "d14" distance of L1.start L1.end
  measures "d15" distance of L1.end L2.end
  measures "d16" distance of L1.end L4.end
extrude "Extrude3" add sketch "Sketch3" against normal blind 3 contours A1 L0 A2 L1 L2 L3 | A1 L0 A2 L1 L4 L5 | A1 L7 L8 L9 L10
fillet "Fillet3" radius 4 8 edges at (45, 5, 1.5) (45, -5, 1.5) (34.641, 5, 1.5) (34.641, -5, 1.5) (-34.641, -5, 1.5) (-45, -5, 1.5) (-45, 5, 1.5) (-34.641, 5, 1.5)
fillet "Fillet4" radius 3 2 edges at (-35, 0, 3) (35, 0, 3)
fillet "Fillet5" radius 1 37 edges at (35.197, 6.0956, 4.0491) (37.8077, 5.0024, 3) (39.4737, 5, 3) (43.8284, 3.8284, 3) (45, 0, 3) (43.8284, -3.8284, 3) (39.4737, -5, 3) (37.8077, -5.0024, 3) (35.1967, -6.0958, 4.0493) (35.4666, 5.8621, 0) (0, 35, 0) (-35.4666, 5.8621, 0) (-39.4737, 5, 0) (-43.8284, 3.8284, 0) (-45, 0, 0) (-43.8284, -3.8284, 0) (-39.4737, -5, 0) (-35.4666, -5.8621, 0) (0, -35, 0) (35.4666, -5.8621, 0) (39.4737, -5, 0) (43.8284, -3.8284, 0) (45, 0, 0) (43.8284, 3.8284, 0) (39.4737, 5, 0) (-35.197, -6.0956, 4.0491) (-37.8077, -5.0024, 3) (-39.4737, -5, 3) (-43.8284, -3.8284, 3) (-45, 0, 3) (-43.8284, 3.8284, 3) (-39.4737, 5, 3) (-37.8077, 5.0024, 3) (-35.1967, 6.0958, 4.0493) (-29.8345, 11.5717, 0) (21.4435, -8.3172, 38) (21.4435, 8.3172, 35)

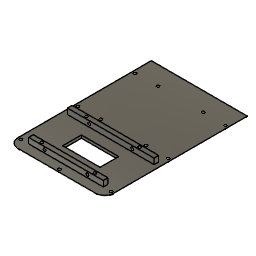
design "baseplate2"
Autodesk Fusion 360 part; units mm, degrees
sketch "Sketch1" plane through (0, 0, 0) normal (0, 0, 1) x (1, 0, 0)
  line L0 (0, 0) -> (-51.5, 0)
  line L1 (0, 0) -> (51.5, 0)
  line L2 (-51.5, 0) -> (-51.5, 265)
  line L3 (-51.5, 265) -> (51.5, 265)
  line L4 (51.5, 265) -> (51.5, 0)
  dimension "d1" = 51.5
  dimension "d2" = 51.5
  dimension "d3" = 265
  constraint coincident L0.start L1.start
  constraint horizontal L0
  constraint parallel L0 L1
  constraint perpendicular L0 L2
  constraint perpendicular L2 L3
  constraint perpendicular L1 L4
  measures "d1" distance of L0.start L0.end
  measures "d2" distance of L0.start L1.end
  measures "d3" distance of L0.end L2.end
extrude "Extrude1" add sketch "Sketch1" along normal blind 3
sketch "Sketch2" plane through (0, 0, 3) normal (0, 0, 1) x (-1, 0, 0)
  line L0 (51.5, 0) -> (-51.5, 0)
  line L1 (-51.5, 0) -> (-51.5, -265)
  line L2 (-51.5, -265) -> (51.5, -265)
  line L3 (51.5, -265) -> (51.5, 0)
  line L4 (0, 0) -> (0, -10)
  line L5 (0, -10) -> (46.5, -10)
  line L6 (0, -10) -> (-46.5, -10)
  line L7 (46.5, -10) -> (46.5, -15)
  line L8 (-46.5, -10) -> (-46.5, -15)
  line L9 (-46.5, -15) -> (46.5, -15)
  line L10 (0, -15) -> (0, -58)
  line L11 (0, -36.5) -> (25, -36.5)
  line L12 (-46.5, -58) -> (46.5, -58)
  line L13 (0, -63) -> (46.5, -63)
  line L14 (0, -63) -> (-46.5, -63)
  line L15 (46.5, -63) -> (46.5, -58)
  line L16 (-46.5, -63) -> (-46.5, -58)
  dimension "d6" = 10
  dimension "d7" = 46.5
  dimension "d8" = 46.5
  dimension "d9" = 5
  dimension "d10" = 43
  constraint coincident L4.start origin
  constraint perpendicular L0 L4
  constraint perpendicular L3 L5
  constraint perpendicular L4 L6
  constraint perpendicular L5 L7
  constraint perpendicular L6 L8
  constraint perpendicular L7 L9
  constraint midpoint L9 L10.start
  constraint perpendicular L9 L10
  constraint midpoint L10 L11.start
  constraint perpendicular L10 L11
  constraint symmetric L4.end L11 L13.start
  constraint symmetric L5.end L11 L13.end
  constraint symmetric L6.end L11 L14.end
  constraint symmetric L7.end L11 L12.end
  constraint symmetric L8.end L11 L12.start
  measures "d6" distance of L4.start L4.end
  measures "d7" distance of L4.end L5.end
  measures "d8" distance of L4.end L6.end
  measures "d9" distance of L5.end L7.end
  measures "d10" distance of L10.start L10.end
extrude "Extrude2" add sketch "Sketch2" along normal blind 6 contours L5 L6 L7 L8 L9 | L12 L13 L14 L15 L16
sketch "Sketch3" plane through (0, 10, 0) normal (0, -1, 0) x (1, 0, 0)
  line L0 (-46.5, 3) -> (46.5, 3)
  line L1 (46.5, 3) -> (46.5, 9)
  line L2 (46.5, 9) -> (-46.5, 9)
  line L3 (-46.5, 9) -> (-46.5, 3)
  line L4 (0, 9) -> (0, 6)
  line L5 (0, 6) -> (-23, 6)
  line L6 (0, 6) -> (23, 6)
  circle A0 centre (-23, 6) radius 1.5
  circle A1 centre (23, 6) radius 1.5
  dimension "d13" = 23
  dimension "d14" = 23
  dimension "d15" = 3
  dimension "d16" = 3
  constraint midpoint L2 L4.start
  constraint perpendicular L2 L4
  constraint perpendicular L4 L5
  constraint perpendicular L4 L6
  constraint coincident L5.end A0.centre
  constraint coincident L6.end A1.centre
  measures "d13" distance of L4.end L5.end
  measures "d14" distance of L4.end L6.end
  measures "d15" diameter of A0
  measures "d16" diameter of A1
extrude "Extrude3" cut sketch "Sketch3" against normal blind 53 contours A0 | A1
sketch "Sketch4" plane through (0, 0, 3) normal (0, 0, 1) x (-1, 0, 0)
  line L0 (46.5, -10) -> (46.5, -15)
  line L1 (46.5, -15) -> (-46.5, -15)
  line L2 (-46.5, -15) -> (-46.5, -10)
  line L3 (-46.5, -10) -> (46.5, -10)
  line L4 (-46.5, -63) -> (-46.5, -58)
  line L5 (-46.5, -58) -> (46.5, -58)
  line L6 (46.5, -58) -> (46.5, -63)
  line L7 (46.5, -63) -> (-46.5, -63)
  line L8 (51.5, 0) -> (-51.5, 0)
  line L9 (-51.5, 0) -> (-51.5, -265)
  line L10 (-51.5, -265) -> (51.5, -265)
  line L11 (51.5, -265) -> (51.5, 0)
  line L12 (0, -63) -> (0, -71.5)
  line L13 (-24.25, -71.5) -> (-24.25, -133)
  line L14 (-24.25, -133) -> (24.25, -133)
  line L15 (24.25, -133) -> (24.25, -74.5)
  circle A0 centre (24.25, -71.5) radius 1.5
  circle A1 centre (-24.25, -71.5) radius 1.5
  line L16 (-24.25, -71.5) -> (24.25, -71.5)
  circle A2 centre (-24.25, -133) radius 1.5
  circle A3 centre (24.25, -133) radius 1.5
  point P0 (24.25, -133)
  point P1 (-24.25, -133)
  dimension "d19" = 8.5
  dimension "d20" = 61.5
  dimension "d21" = 48.5
  dimension "d22" = 3
  dimension "d23" = 3
  dimension "d24" = 3
  dimension "d25" = 3
  constraint midpoint L7 L12.start
  constraint perpendicular L7 L12
  constraint perpendicular L13 L14
  constraint perpendicular L14 L15
  constraint coincident L13.start A1.centre
  constraint coincident P1 L13.end
  constraint coincident P0 L14.end
  constraint coincident A0.centre L16.end
  constraint perpendicular L13 L16
  measures "d19" distance of L12.start L12.end
  measures "d20" distance of L13.start P1
  measures "d21" distance of P1 P0
  measures "d22" diameter of A1
  measures "d23" diameter of A0
  measures "d24" diameter of A2
  measures "d25" diameter of A3
extrude "Extrude4" cut sketch "Sketch4" against normal blind 3 contours L13 A1 L16 | L13 A1 L16 | L13 L14 A2 | L13 L14 A2 | L14 L15 A3 | L14 L15 A3 | A0
sketch "Sketch5" plane through (0, 0, 3) normal (0, 0, 1) x (-1, 0, 0)
  circle A0 centre (-24.25, -133) radius 1.5
  circle A1 centre (24.25, -71.5) radius 1.5
  circle A2 centre (24.25, -133) radius 1.5
  circle A3 centre (-24.25, -71.5) radius 1.5
  line L0 (46.5, -10) -> (46.5, -15)
  line L1 (46.5, -15) -> (-46.5, -15)
  line L2 (-46.5, -15) -> (-46.5, -10)
  line L3 (-46.5, -10) -> (46.5, -10)
  line L4 (-46.5, -63) -> (-46.5, -58)
  line L5 (-46.5, -58) -> (46.5, -58)
  line L6 (46.5, -58) -> (46.5, -63)
  line L7 (46.5, -63) -> (-46.5, -63)
  line L8 (51.5, 0) -> (-51.5, 0)
  line L9 (-51.5, 0) -> (-51.5, -265)
  line L10 (-51.5, -265) -> (51.5, -265)
  line L11 (51.5, -265) -> (51.5, 0)
  line L12 (24.25, -133) -> (-24.25, -133)
  line L13 (0, -133) -> (0, -173)
  line L14 (0, -238) -> (-35, -238)
  line L15 (0, -238) -> (35, -238)
  line L16 (0, -233) -> (35, -233)
  line L17 (0, -233) -> (-35, -233)
  line L18 (0, -178) -> (35, -178)
  line L19 (0, -178) -> (-35, -178)
  line L20 (0, -173) -> (-35, -173)
  line L21 (0, -173) -> (35, -173)
  line L22 (-35, -178) -> (-35, -173)
  line L23 (35, -173) -> (35, -178)
  line L24 (35, -238) -> (35, -233)
  line L25 (-35, -238) -> (-35, -233)
  line L26 (0, -173) -> (-12.9802, -153.9099)
  dimension "d28" = 40
  dimension "d29" = 5
  constraint coincident A2.centre L12.start
  constraint coincident A0.centre L12.end
  constraint midpoint L12 L13.start
  constraint perpendicular L12 L13
  constraint perpendicular L20 L22
  constraint perpendicular L3 L23
  constraint perpendicular L16 L24
  constraint perpendicular L17 L25
  measures "d28" distance of L13.start L13.end
  measures "d29" distance of L13.end L18.start
extrude "Extrude5" add sketch "Sketch5" along normal blind 10 contours L14 L15 L16 L17 L24 L25 | L18 L19 L20 L21 L22 L23
sketch "Sketch6" plane through (0, 238, 0) normal (0, 1, 0) x (-1, 0, 0)
  line L0 (-35, 3) -> (35, 3)
  line L1 (35, 3) -> (35, 13)
  line L2 (35, 13) -> (-35, 13)
  line L3 (-35, 13) -> (-35, 3)
  line L4 (0, 13) -> (0, 3)
  line L5 (0, 8) -> (-22.5, 8)
  line L6 (0, 8) -> (22.5, 8)
  circle A0 centre (-22.5, 8) radius 2
  circle A1 centre (22.5, 8) radius 2
  dimension "d32" = 22.5
  dimension "d33" = 22.5
  dimension "d34" = 4
  dimension "d35" = 4
  constraint midpoint L2 L4.start
  constraint midpoint L0 L4.end
  constraint midpoint L4 L5.start
  constraint perpendicular L4 L5
  constraint perpendicular L4 L6
  constraint coincident L5.end A0.centre
  constraint coincident L6.end A1.centre
  measures "d32" distance of L5.start L5.end
  measures "d33" distance of L5.start L6.end
  measures "d34" diameter of A0
  measures "d35" diameter of A1
extrude "Extrude6" cut sketch "Sketch6" against normal blind 80 contours A0 | A1